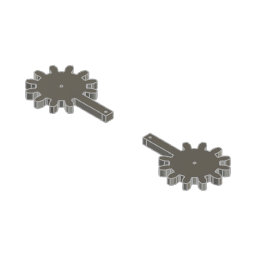
arm_gears v1 (Autodesk Fusion 360 design; units mm, degrees)
description: Spur Gear; Module: 5.0; Num Teeth: 12; Pressure Angle: 14.500000000000002; Backlash: 0.00 mm
Autodesk Fusion 360 part; units mm, degrees
(part 1 of 2)
sketch "スケッチ1" plane through (0, 0, 0) normal (0, 0, 1) x (1, 0, 0) in component "Spur Gear (12 teeth)"
  circle A0 centre (0, 0) radius 23.9492
  circle A1 centre (0, 0) radius 1.5
extrude "押し出し1" add sketch "スケッチ1" along normal blind 8 makes body 1 in component "Spur Gear (12 teeth)"
sketch "スケッチ2" plane through (0, 0, 0) normal (0, 0, 1) x (1, 0, 0) in component "Spur Gear (12 teeth)"
  spline S0 degree 5 poles (28.7745, -3.9507) (28.792, -3.9531) (28.8272, -3.9574) (28.88, -3.9623) (28.9507, -3.9658) (29.0393, -3.9662) (29.1282, -3.9638) (29.2172, -3.9595) (29.3063, -3.9544) (29.3954, -3.9485) (29.4846, -3.9419) (29.5738, -3.9345) (29.663, -3.9257) (29.7523, -3.9156) (29.8417, -3.904) (29.9311, -3.8911) (30.0205, -3.8771) (30.11, -3.8622) (30.1994, -3.8464) (30.2888, -3.8299) (30.3782, -3.8126) (30.4676, -3.7945) (30.557, -3.7754) (30.6464, -3.7555) (30.7357, -3.7347) (30.8251, -3.7131) (30.9144, -3.6907) (31.0037, -3.6675) (31.0929, -3.6435) (31.1821, -3.6189) (31.2712, -3.5935) (31.3604, -3.5674) (31.4494, -3.5406) (31.5384, -3.5131) (31.6274, -3.4848) (31.7163, -3.4559) (31.8051, -3.4263) (31.8939, -3.396) (31.9826, -3.365) (32.0713, -3.3335) (32.1598, -3.3012) (32.2484, -3.2683) (32.3368, -3.2348) (32.4251, -3.2007) (32.5134, -3.1659) (32.6016, -3.1305) (32.6897, -3.0945) (32.7778, -3.0579) (32.8657, -3.0207) (32.9536, -2.9829) (33.0413, -2.9445) (33.129, -2.9056) (33.2166, -2.866) (33.3041, -2.8259) (33.3915, -2.7852) (33.4787, -2.7439) (33.5659, -2.7021) (33.653, -2.6597) (33.7399, -2.6167) (33.8268, -2.5732) (33.9135, -2.5292) (34.0002, -2.4846) (34.0867, -2.4394) (34.1731, -2.3938) (34.2594, -2.3476) (34.3455, -2.3008) (34.4316, -2.2536) (34.5175, -2.2058) (34.6033, -2.1575) (34.6889, -2.1087) (34.7745, -2.0593) (34.8428, -2.0194) (34.894, -1.9893) (34.9281, -1.9691) (34.9451, -1.959) knots 0 0 0 0 0 0 0.01428571 0.02857143 0.04285714 0.05714286 0.07142857 0.08571429 0.1 0.11428571 0.12857143 0.14285714 0.15714286 0.17142857 0.18571429 0.2 0.21428571 0.22857143 0.24285714 0.25714286 0.27142857 0.28571429 0.3 0.31428571 0.32857143 0.34285714 0.35714286 0.37142857 0.38571429 0.4 0.41428571 0.42857143 0.44285714 0.45714286 0.47142857 0.48571429 0.5 0.51428571 0.52857143 0.54285714 0.55714286 0.57142857 0.58571429 0.6 0.61428571 0.62857143 0.64285714 0.65714286 0.67142857 0.68571429 0.7 0.71428571 0.72857143 0.74285714 0.75714286 0.77142857 0.78571429 0.8 0.81428571 0.82857143 0.84285714 0.85714286 0.87142857 0.88571429 0.9 0.91428571 0.92857143 0.94285714 0.95714286 0.97142857 0.98571429 1 1 1 1 1 1
  spline S1 degree 5 poles (28.7745, 3.9507) (28.792, 3.9531) (28.8272, 3.9574) (28.88, 3.9623) (28.9507, 3.9658) (29.0393, 3.9662) (29.1282, 3.9638) (29.2172, 3.9595) (29.3063, 3.9544) (29.3954, 3.9485) (29.4846, 3.9419) (29.5738, 3.9345) (29.663, 3.9257) (29.7523, 3.9156) (29.8417, 3.904) (29.9311, 3.8911) (30.0205, 3.8771) (30.11, 3.8622) (30.1994, 3.8464) (30.2888, 3.8299) (30.3782, 3.8126) (30.4676, 3.7945) (30.557, 3.7754) (30.6464, 3.7555) (30.7357, 3.7347) (30.8251, 3.7131) (30.9144, 3.6907) (31.0037, 3.6675) (31.0929, 3.6435) (31.1821, 3.6189) (31.2712, 3.5935) (31.3604, 3.5674) (31.4494, 3.5406) (31.5384, 3.5131) (31.6274, 3.4848) (31.7163, 3.4559) (31.8051, 3.4263) (31.8939, 3.396) (31.9826, 3.365) (32.0713, 3.3335) (32.1598, 3.3012) (32.2484, 3.2683) (32.3368, 3.2348) (32.4251, 3.2007) (32.5134, 3.1659) (32.6016, 3.1305) (32.6897, 3.0945) (32.7778, 3.0579) (32.8657, 3.0207) (32.9536, 2.9829) (33.0413, 2.9445) (33.129, 2.9056) (33.2166, 2.866) (33.3041, 2.8259) (33.3915, 2.7852) (33.4787, 2.7439) (33.5659, 2.7021) (33.653, 2.6597) (33.7399, 2.6167) (33.8268, 2.5732) (33.9135, 2.5292) (34.0002, 2.4846) (34.0867, 2.4394) (34.1731, 2.3938) (34.2594, 2.3476) (34.3455, 2.3008) (34.4316, 2.2536) (34.5175, 2.2058) (34.6033, 2.1575) (34.6889, 2.1087) (34.7745, 2.0593) (34.8428, 2.0194) (34.894, 1.9893) (34.9281, 1.9691) (34.9451, 1.959) knots 0 0 0 0 0 0 0.01428571 0.02857143 0.04285714 0.05714286 0.07142857 0.08571429 0.1 0.11428571 0.12857143 0.14285714 0.15714286 0.17142857 0.18571429 0.2 0.21428571 0.22857143 0.24285714 0.25714286 0.27142857 0.28571429 0.3 0.31428571 0.32857143 0.34285714 0.35714286 0.37142857 0.38571429 0.4 0.41428571 0.42857143 0.44285714 0.45714286 0.47142857 0.48571429 0.5 0.51428571 0.52857143 0.54285714 0.55714286 0.57142857 0.58571429 0.6 0.61428571 0.62857143 0.64285714 0.65714286 0.67142857 0.68571429 0.7 0.71428571 0.72857143 0.74285714 0.75714286 0.77142857 0.78571429 0.8 0.81428571 0.82857143 0.84285714 0.85714286 0.87142857 0.88571429 0.9 0.91428571 0.92857143 0.94285714 0.95714286 0.97142857 0.98571429 1 1 1 1 1 1
  arc A0 (34.9451, -1.959) -> (34.9451, 1.959) centre (0, 0) ccw
  line L0 (23.7167, -3.2576) -> (28.7745, -3.9507)
  line L1 (23.7167, 3.2576) -> (28.7745, 3.9507)
  line L2 (23.7167, -3.2576) -> (23.7167, 3.2576)
  point P0 (29.2025, -3.9601)
  point P1 (29.636, -3.9282)
  point P2 (30.0729, -3.8683)
  point P3 (30.5122, -3.7849)
  point P4 (30.9534, -3.6804)
  point P5 (31.396, -3.5566)
  point P6 (31.8397, -3.4144)
  point P7 (32.284, -3.2548)
  point P8 (32.7286, -3.0783)
  point P9 (33.1731, -2.8856)
  point P10 (33.6174, -2.6769)
  point P11 (34.061, -2.4528)
  point P12 (34.5037, -2.2134)
  point P13 (29.2025, 3.9601)
  point P14 (29.636, 3.9282)
  point P15 (30.0729, 3.8683)
  point P16 (30.5122, 3.7849)
  point P17 (30.9534, 3.6804)
  point P18 (31.396, 3.5566)
  point P19 (31.8397, 3.4144)
  point P20 (32.284, 3.2548)
  point P21 (32.7286, 3.0783)
  point P22 (33.1731, 2.8856)
  point P23 (33.6174, 2.6769)
  point P24 (34.061, 2.4528)
  point P25 (34.5037, 2.2134)
extrude "押し出し2" add sketch "スケッチ2" along normal blind 8 bodies 1 in component "Spur Gear (12 teeth)"
fillet "フィレット1" radius 1 2 edges at (23.7264, -3.2589, 4) (23.7264, 3.2589, 4) on bodies 1 in component "Spur Gear (12 teeth)"
pattern_circular "C パターン1" count 12 over 360 about axis through (0, 0, 0) along (0, 0, 1) of "押し出し2", "フィレット1" in component "Spur Gear (12 teeth)"
sketch "スケッチ3" plane through (0, 0, 0) normal (0, 0, 1) x (1, 0, 0) in component "Spur Gear (12 teeth)"
  circle A0 centre (0, 0) radius 30 construction
sketch "スケッチ1 (2)" plane through (0, 0, 8) normal (0, 0, 1) x (-1, 0, 0)
  arc A0 (-22.5216, 8.145) -> (-23.5768, 4.207) centre (0, 0) ccw
  arc A1 (-24.697, 3.3919) -> (-23.5768, 4.207) centre (-24.5612, 4.3827) ccw
  line L0 (-24.697, 3.3919) -> (-28.7745, 3.9507)
  spline S0 degree 5 poles (-28.7745, 3.9507) (-28.792, 3.9531) (-28.8272, 3.9574) (-28.88, 3.9623) (-28.9507, 3.9658) (-29.0393, 3.9662) (-29.1282, 3.9638) (-29.2172, 3.9595) (-29.3063, 3.9544) (-29.3954, 3.9485) (-29.4846, 3.9419) (-29.5738, 3.9345) (-29.663, 3.9257) (-29.7523, 3.9156) (-29.8417, 3.904) (-29.9311, 3.8911) (-30.0205, 3.8771) (-30.11, 3.8622) (-30.1994, 3.8464) (-30.2888, 3.8299) (-30.3782, 3.8126) (-30.4676, 3.7945) (-30.557, 3.7754) (-30.6464, 3.7555) (-30.7357, 3.7347) (-30.8251, 3.7131) (-30.9144, 3.6907) (-31.0037, 3.6675) (-31.0929, 3.6435) (-31.1821, 3.6189) (-31.2712, 3.5935) (-31.3604, 3.5674) (-31.4494, 3.5406) (-31.5384, 3.5131) (-31.6274, 3.4848) (-31.7163, 3.4559) (-31.8051, 3.4263) (-31.8939, 3.396) (-31.9826, 3.365) (-32.0713, 3.3335) (-32.1598, 3.3012) (-32.2484, 3.2683) (-32.3368, 3.2348) (-32.4251, 3.2007) (-32.5134, 3.1659) (-32.6016, 3.1305) (-32.6897, 3.0945) (-32.7778, 3.0579) (-32.8657, 3.0207) (-32.9536, 2.9829) (-33.0413, 2.9445) (-33.129, 2.9056) (-33.2166, 2.866) (-33.3041, 2.8259) (-33.3915, 2.7852) (-33.4787, 2.7439) (-33.5659, 2.7021) (-33.653, 2.6597) (-33.7399, 2.6167) (-33.8268, 2.5732) (-33.9135, 2.5292) (-34.0002, 2.4846) (-34.0867, 2.4394) (-34.1731, 2.3938) (-34.2594, 2.3476) (-34.3455, 2.3008) (-34.4316, 2.2536) (-34.5175, 2.2058) (-34.6033, 2.1575) (-34.6889, 2.1087) (-34.7745, 2.0593) (-34.8428, 2.0194) (-34.894, 1.9893) (-34.9281, 1.9691) (-34.9451, 1.959) knots 0 0 0 0 0 0 0.01428571 0.02857143 0.04285714 0.05714286 0.07142857 0.08571429 0.1 0.11428571 0.12857143 0.14285714 0.15714286 0.17142857 0.18571429 0.2 0.21428571 0.22857143 0.24285714 0.25714286 0.27142857 0.28571429 0.3 0.31428571 0.32857143 0.34285714 0.35714286 0.37142857 0.38571429 0.4 0.41428571 0.42857143 0.44285714 0.45714286 0.47142857 0.48571429 0.5 0.51428571 0.52857143 0.54285714 0.55714286 0.57142857 0.58571429 0.6 0.61428571 0.62857143 0.64285714 0.65714286 0.67142857 0.68571429 0.7 0.71428571 0.72857143 0.74285714 0.75714286 0.77142857 0.78571429 0.8 0.81428571 0.82857143 0.84285714 0.85714286 0.87142857 0.88571429 0.9 0.91428571 0.92857143 0.94285714 0.95714286 0.97142857 0.98571429 1 1 1 1 1 1
  arc A2 (-34.9451, 1.959) -> (-34.9451, -1.959) centre (0, 0) ccw
  spline S1 degree 5 poles (-34.9451, -1.959) (-34.9281, -1.9691) (-34.894, -1.9893) (-34.8428, -2.0194) (-34.7745, -2.0593) (-34.6889, -2.1087) (-34.6033, -2.1575) (-34.5175, -2.2058) (-34.4316, -2.2536) (-34.3455, -2.3008) (-34.2594, -2.3476) (-34.1731, -2.3938) (-34.0867, -2.4394) (-34.0002, -2.4846) (-33.9135, -2.5292) (-33.8268, -2.5732) (-33.7399, -2.6167) (-33.653, -2.6597) (-33.5659, -2.7021) (-33.4787, -2.7439) (-33.3915, -2.7852) (-33.3041, -2.8259) (-33.2166, -2.866) (-33.129, -2.9056) (-33.0413, -2.9445) (-32.9536, -2.9829) (-32.8657, -3.0207) (-32.7778, -3.0579) (-32.6897, -3.0945) (-32.6016, -3.1305) (-32.5134, -3.1659) (-32.4251, -3.2007) (-32.3368, -3.2348) (-32.2484, -3.2683) (-32.1598, -3.3012) (-32.0713, -3.3335) (-31.9826, -3.365) (-31.8939, -3.396) (-31.8051, -3.4263) (-31.7163, -3.4559) (-31.6274, -3.4848) (-31.5384, -3.5131) (-31.4494, -3.5406) (-31.3604, -3.5674) (-31.2712, -3.5935) (-31.1821, -3.6189) (-31.0929, -3.6435) (-31.0037, -3.6675) (-30.9144, -3.6907) (-30.8251, -3.7131) (-30.7357, -3.7347) (-30.6464, -3.7555) (-30.557, -3.7754) (-30.4676, -3.7945) (-30.3782, -3.8126) (-30.2888, -3.8299) (-30.1994, -3.8464) (-30.11, -3.8622) (-30.0205, -3.8771) (-29.9311, -3.8911) (-29.8417, -3.904) (-29.7523, -3.9156) (-29.663, -3.9257) (-29.5738, -3.9345) (-29.4846, -3.9419) (-29.3954, -3.9485) (-29.3063, -3.9544) (-29.2172, -3.9595) (-29.1282, -3.9638) (-29.0393, -3.9662) (-28.9507, -3.9658) (-28.88, -3.9623) (-28.8272, -3.9574) (-28.792, -3.9531) (-28.7745, -3.9507) knots -1 -1 -1 -1 -1 -1 -0.98571429 -0.97142857 -0.95714286 -0.94285714 -0.92857143 -0.91428571 -0.9 -0.88571429 -0.87142857 -0.85714286 -0.84285714 -0.82857143 -0.81428571 -0.8 -0.78571429 -0.77142857 -0.75714286 -0.74285714 -0.72857143 -0.71428571 -0.7 -0.68571429 -0.67142857 -0.65714286 -0.64285714 -0.62857143 -0.61428571 -0.6 -0.58571429 -0.57142857 -0.55714286 -0.54285714 -0.52857143 -0.51428571 -0.5 -0.48571429 -0.47142857 -0.45714286 -0.44285714 -0.42857143 -0.41428571 -0.4 -0.38571429 -0.37142857 -0.35714286 -0.34285714 -0.32857143 -0.31428571 -0.3 -0.28571429 -0.27142857 -0.25714286 -0.24285714 -0.22857143 -0.21428571 -0.2 -0.18571429 -0.17142857 -0.15714286 -0.14285714 -0.12857143 -0.11428571 -0.1 -0.08571429 -0.07142857 -0.05714286 -0.04285714 -0.02857143 -0.01428571 0 0 0 0 0 0
  line L1 (-28.7745, -3.9507) -> (-24.697, -3.3919)
  arc A3 (-23.5768, -4.207) -> (-24.697, -3.3919) centre (-24.5612, -4.3827) ccw
  arc A4 (-23.5768, -4.207) -> (-22.5216, -8.145) centre (0, 0) ccw
  arc A5 (-23.0842, -9.411) -> (-22.5216, -8.145) centre (-23.462, -8.4851) ccw
  line L2 (-23.0842, -9.411) -> (-26.8948, -10.9659)
  spline S2 degree 5 poles (-26.8948, -10.9659) (-26.9112, -10.9726) (-26.9438, -10.9864) (-26.992, -11.0086) (-27.055, -11.0409) (-27.1319, -11.0848) (-27.2076, -11.1314) (-27.2826, -11.1795) (-27.3571, -11.2286) (-27.4314, -11.2782) (-27.5053, -11.3285) (-27.5789, -11.3795) (-27.6518, -11.4317) (-27.7241, -11.4852) (-27.7957, -11.5399) (-27.8667, -11.5957) (-27.9371, -11.6526) (-28.0071, -11.7102) (-28.0767, -11.7686) (-28.1458, -11.8276) (-28.2146, -11.8873) (-28.283, -11.9477) (-28.3509, -12.0089) (-28.4183, -12.0708) (-28.4853, -12.1335) (-28.5519, -12.1969) (-28.618, -12.261) (-28.6837, -12.3257) (-28.749, -12.3911) (-28.8139, -12.457) (-28.8784, -12.5236) (-28.9426, -12.5907) (-29.0063, -12.6585) (-29.0696, -12.7268) (-29.1325, -12.7958) (-29.195, -12.8653) (-29.2572, -12.9353) (-29.3189, -13.0059) (-29.3803, -13.0771) (-29.4413, -13.1488) (-29.5019, -13.221) (-29.5621, -13.2937) (-29.6219, -13.367) (-29.6813, -13.4407) (-29.7404, -13.515) (-29.7991, -13.5897) (-29.8574, -13.6649) (-29.9154, -13.7406) (-29.9729, -13.8168) (-30.0301, -13.8935) (-30.0869, -13.9706) (-30.1434, -14.0482) (-30.1994, -14.1263) (-30.2551, -14.2048) (-30.3104, -14.2837) (-30.3654, -14.3631) (-30.42, -14.4429) (-30.4742, -14.5231) (-30.528, -14.6038) (-30.5815, -14.6849) (-30.6346, -14.7664) (-30.6873, -14.8484) (-30.7397, -14.9307) (-30.7916, -15.0135) (-30.8433, -15.0966) (-30.8945, -15.1802) (-30.9454, -15.2641) (-30.9959, -15.3485) (-31.0461, -15.4332) (-31.0958, -15.5183) (-31.1452, -15.6038) (-31.1845, -15.6725) (-31.2137, -15.7242) (-31.2332, -15.7587) (-31.2429, -15.776) knots 0 0 0 0 0 0 0.01428571 0.02857143 0.04285714 0.05714286 0.07142857 0.08571429 0.1 0.11428571 0.12857143 0.14285714 0.15714286 0.17142857 0.18571429 0.2 0.21428571 0.22857143 0.24285714 0.25714286 0.27142857 0.28571429 0.3 0.31428571 0.32857143 0.34285714 0.35714286 0.37142857 0.38571429 0.4 0.41428571 0.42857143 0.44285714 0.45714286 0.47142857 0.48571429 0.5 0.51428571 0.52857143 0.54285714 0.55714286 0.57142857 0.58571429 0.6 0.61428571 0.62857143 0.64285714 0.65714286 0.67142857 0.68571429 0.7 0.71428571 0.72857143 0.74285714 0.75714286 0.77142857 0.78571429 0.8 0.81428571 0.82857143 0.84285714 0.85714286 0.87142857 0.88571429 0.9 0.91428571 0.92857143 0.94285714 0.95714286 0.97142857 0.98571429 1 1 1 1 1 1
  arc A6 (-31.2429, -15.776) -> (-29.2839, -19.1691) centre (0, 0) ccw
  spline S3 degree 5 poles (-29.2839, -19.1691) (-29.2641, -19.1693) (-29.2244, -19.1698) (-29.165, -19.1703) (-29.0859, -19.1707) (-28.9872, -19.1706) (-28.8886, -19.1701) (-28.7901, -19.169) (-28.6918, -19.1674) (-28.5937, -19.1653) (-28.4957, -19.1627) (-28.3979, -19.1596) (-28.3002, -19.156) (-28.2027, -19.1518) (-28.1054, -19.1471) (-28.0082, -19.1419) (-27.9113, -19.1361) (-27.8145, -19.1298) (-27.7179, -19.123) (-27.6215, -19.1157) (-27.5253, -19.1078) (-27.4292, -19.0993) (-27.3334, -19.0903) (-27.2378, -19.0808) (-27.1424, -19.0707) (-27.0472, -19.0601) (-26.9522, -19.0489) (-26.8574, -19.0371) (-26.7629, -19.0248) (-26.6686, -19.0119) (-26.5745, -18.9985) (-26.4807, -18.9844) (-26.3871, -18.9698) (-26.2937, -18.9546) (-26.2006, -18.9389) (-26.1078, -18.9225) (-26.0152, -18.9055) (-25.9229, -18.888) (-25.8309, -18.8698) (-25.7392, -18.851) (-25.6477, -18.8316) (-25.5565, -18.8116) (-25.4657, -18.7909) (-25.3752, -18.7696) (-25.2849, -18.7477) (-25.1951, -18.7251) (-25.1055, -18.7018) (-25.0162, -18.6779) (-24.9273, -18.6534) (-24.8388, -18.6282) (-24.7506, -18.6022) (-24.6628, -18.5756) (-24.5754, -18.5481) (-24.4885, -18.5199) (-24.402, -18.4909) (-24.3159, -18.4612) (-24.2302, -18.4308) (-24.1449, -18.3997) (-24.06, -18.3679) (-23.9755, -18.3354) (-23.8917, -18.3018) (-23.8085, -18.2672) (-23.7261, -18.2313) (-23.6444, -18.1942) (-23.5634, -18.1561) (-23.4829, -18.1172) (-23.4028, -18.0777) (-23.3231, -18.0377) (-23.2439, -17.9968) (-23.1657, -17.9545) (-23.0891, -17.9099) (-23.0297, -17.8714) (-22.9864, -17.8408) (-22.9581, -17.8195) (-22.9441, -17.8086) knots -1 -1 -1 -1 -1 -1 -0.98571429 -0.97142857 -0.95714286 -0.94285714 -0.92857143 -0.91428571 -0.9 -0.88571429 -0.87142857 -0.85714286 -0.84285714 -0.82857143 -0.81428571 -0.8 -0.78571429 -0.77142857 -0.75714286 -0.74285714 -0.72857143 -0.71428571 -0.7 -0.68571429 -0.67142857 -0.65714286 -0.64285714 -0.62857143 -0.61428571 -0.6 -0.58571429 -0.57142857 -0.55714286 -0.54285714 -0.52857143 -0.51428571 -0.5 -0.48571429 -0.47142857 -0.45714286 -0.44285714 -0.42857143 -0.41428571 -0.4 -0.38571429 -0.37142857 -0.35714286 -0.34285714 -0.32857143 -0.31428571 -0.3 -0.28571429 -0.27142857 -0.25714286 -0.24285714 -0.22857143 -0.21428571 -0.2 -0.18571429 -0.17142857 -0.15714286 -0.14285714 -0.12857143 -0.11428571 -0.1 -0.08571429 -0.07142857 -0.05714286 -0.04285714 -0.02857143 -0.01428571 0 0 0 0 0 0
  line L3 (-22.9441, -17.8086) -> (-19.6923, -15.286)
  arc A7 (-18.3146, -15.4318) -> (-19.6923, -15.286) centre (-19.0793, -16.0761) ccw
  arc A8 (-18.3146, -15.4318) -> (-15.4318, -18.3146) centre (0, 0) ccw
  arc A9 (-15.286, -19.6923) -> (-15.4318, -18.3146) centre (-16.0761, -19.0793) ccw
  line L4 (-15.286, -19.6923) -> (-17.8086, -22.9441)
  spline S4 degree 5 poles (-17.8086, -22.9441) (-17.8195, -22.9581) (-17.8408, -22.9864) (-17.8714, -23.0297) (-17.9099, -23.0891) (-17.9545, -23.1657) (-17.9968, -23.2439) (-18.0377, -23.3231) (-18.0777, -23.4028) (-18.1172, -23.4829) (-18.1561, -23.5634) (-18.1942, -23.6444) (-18.2313, -23.7261) (-18.2672, -23.8085) (-18.3018, -23.8917) (-18.3354, -23.9755) (-18.3679, -24.06) (-18.3997, -24.1449) (-18.4308, -24.2302) (-18.4612, -24.3159) (-18.4909, -24.402) (-18.5199, -24.4885) (-18.5481, -24.5754) (-18.5756, -24.6628) (-18.6022, -24.7506) (-18.6282, -24.8388) (-18.6534, -24.9273) (-18.6779, -25.0162) (-18.7018, -25.1055) (-18.7251, -25.1951) (-18.7477, -25.2849) (-18.7696, -25.3752) (-18.7909, -25.4657) (-18.8116, -25.5565) (-18.8316, -25.6477) (-18.851, -25.7392) (-18.8698, -25.8309) (-18.888, -25.9229) (-18.9055, -26.0152) (-18.9225, -26.1078) (-18.9389, -26.2006) (-18.9546, -26.2937) (-18.9698, -26.3871) (-18.9844, -26.4807) (-18.9985, -26.5745) (-19.0119, -26.6686) (-19.0248, -26.7629) (-19.0371, -26.8574) (-19.0489, -26.9522) (-19.0601, -27.0472) (-19.0707, -27.1424) (-19.0808, -27.2378) (-19.0903, -27.3334) (-19.0993, -27.4292) (-19.1078, -27.5253) (-19.1157, -27.6215) (-19.123, -27.7179) (-19.1298, -27.8145) (-19.1361, -27.9113) (-19.1419, -28.0082) (-19.1471, -28.1054) (-19.1518, -28.2027) (-19.156, -28.3002) (-19.1596, -28.3979) (-19.1627, -28.4957) (-19.1653, -28.5937) (-19.1674, -28.6918) (-19.169, -28.7901) (-19.1701, -28.8886) (-19.1706, -28.9872) (-19.1707, -29.0859) (-19.1703, -29.165) (-19.1698, -29.2244) (-19.1693, -29.2641) (-19.1691, -29.2839) knots 0 0 0 0 0 0 0.01428571 0.02857143 0.04285714 0.05714286 0.07142857 0.08571429 0.1 0.11428571 0.12857143 0.14285714 0.15714286 0.17142857 0.18571429 0.2 0.21428571 0.22857143 0.24285714 0.25714286 0.27142857 0.28571429 0.3 0.31428571 0.32857143 0.34285714 0.35714286 0.37142857 0.38571429 0.4 0.41428571 0.42857143 0.44285714 0.45714286 0.47142857 0.48571429 0.5 0.51428571 0.52857143 0.54285714 0.55714286 0.57142857 0.58571429 0.6 0.61428571 0.62857143 0.64285714 0.65714286 0.67142857 0.68571429 0.7 0.71428571 0.72857143 0.74285714 0.75714286 0.77142857 0.78571429 0.8 0.81428571 0.82857143 0.84285714 0.85714286 0.87142857 0.88571429 0.9 0.91428571 0.92857143 0.94285714 0.95714286 0.97142857 0.98571429 1 1 1 1 1 1
  arc A10 (-19.1691, -29.2839) -> (-15.776, -31.2429) centre (0, 0) ccw
  spline S5 degree 5 poles (-15.776, -31.2429) (-15.7587, -31.2332) (-15.7242, -31.2137) (-15.6725, -31.1845) (-15.6038, -31.1452) (-15.5183, -31.0958) (-15.4332, -31.0461) (-15.3485, -30.9959) (-15.2641, -30.9454) (-15.1802, -30.8945) (-15.0966, -30.8433) (-15.0135, -30.7916) (-14.9307, -30.7397) (-14.8484, -30.6873) (-14.7664, -30.6346) (-14.6849, -30.5815) (-14.6038, -30.528) (-14.5231, -30.4742) (-14.4429, -30.42) (-14.3631, -30.3654) (-14.2837, -30.3104) (-14.2048, -30.2551) (-14.1263, -30.1994) (-14.0482, -30.1434) (-13.9706, -30.0869) (-13.8935, -30.0301) (-13.8168, -29.9729) (-13.7406, -29.9154) (-13.6649, -29.8574) (-13.5897, -29.7991) (-13.515, -29.7404) (-13.4407, -29.6813) (-13.367, -29.6219) (-13.2937, -29.5621) (-13.221, -29.5019) (-13.1488, -29.4413) (-13.0771, -29.3803) (-13.0059, -29.3189) (-12.9353, -29.2572) (-12.8653, -29.195) (-12.7958, -29.1325) (-12.7268, -29.0696) (-12.6585, -29.0063) (-12.5907, -28.9426) (-12.5236, -28.8784) (-12.457, -28.8139) (-12.3911, -28.749) (-12.3257, -28.6837) (-12.261, -28.618) (-12.1969, -28.5519) (-12.1335, -28.4853) (-12.0708, -28.4183) (-12.0089, -28.3509) (-11.9477, -28.283) (-11.8873, -28.2146) (-11.8276, -28.1458) (-11.7686, -28.0767) (-11.7102, -28.0071) (-11.6526, -27.9371) (-11.5957, -27.8667) (-11.5399, -27.7957) (-11.4852, -27.7241) (-11.4317, -27.6518) (-11.3795, -27.5789) (-11.3285, -27.5053) (-11.2782, -27.4314) (-11.2286, -27.3571) (-11.1795, -27.2826) (-11.1314, -27.2076) (-11.0848, -27.1319) (-11.0409, -27.055) (-11.0086, -26.992) (-10.9864, -26.9438) (-10.9726, -26.9112) (-10.9659, -26.8948) knots -1 -1 -1 -1 -1 -1 -0.98571429 -0.97142857 -0.95714286 -0.94285714 -0.92857143 -0.91428571 -0.9 -0.88571429 -0.87142857 -0.85714286 -0.84285714 -0.82857143 -0.81428571 -0.8 -0.78571429 -0.77142857 -0.75714286 -0.74285714 -0.72857143 -0.71428571 -0.7 -0.68571429 -0.67142857 -0.65714286 -0.64285714 -0.62857143 -0.61428571 -0.6 -0.58571429 -0.57142857 -0.55714286 -0.54285714 -0.52857143 -0.51428571 -0.5 -0.48571429 -0.47142857 -0.45714286 -0.44285714 -0.42857143 -0.41428571 -0.4 -0.38571429 -0.37142857 -0.35714286 -0.34285714 -0.32857143 -0.31428571 -0.3 -0.28571429 -0.27142857 -0.25714286 -0.24285714 -0.22857143 -0.21428571 -0.2 -0.18571429 -0.17142857 -0.15714286 -0.14285714 -0.12857143 -0.11428571 -0.1 -0.08571429 -0.07142857 -0.05714286 -0.04285714 -0.02857143 -0.01428571 0 0 0 0 0 0
  line L5 (-10.9659, -26.8948) -> (-9.411, -23.0842)
  arc A11 (-8.145, -22.5216) -> (-9.411, -23.0842) centre (-8.4851, -23.462) ccw
  arc A12 (-8.145, -22.5216) -> (-4.207, -23.5768) centre (0, 0) ccw
  arc A13 (-3.3919, -24.697) -> (-4.207, -23.5768) centre (-4.3827, -24.5612) ccw
  line L6 (-3.3919, -24.697) -> (-3.9507, -28.7745)
  spline S6 degree 5 poles (-3.9507, -28.7745) (-3.9531, -28.792) (-3.9574, -28.8272) (-3.9623, -28.88) (-3.9658, -28.9507) (-3.9662, -29.0393) (-3.9638, -29.1282) (-3.9595, -29.2172) (-3.9544, -29.3063) (-3.9485, -29.3954) (-3.9419, -29.4846) (-3.9345, -29.5738) (-3.9257, -29.663) (-3.9156, -29.7523) (-3.904, -29.8417) (-3.8911, -29.9311) (-3.8771, -30.0205) (-3.8622, -30.11) (-3.8464, -30.1994) (-3.8299, -30.2888) (-3.8126, -30.3782) (-3.7945, -30.4676) (-3.7754, -30.557) (-3.7555, -30.6464) (-3.7347, -30.7357) (-3.7131, -30.8251) (-3.6907, -30.9144) (-3.6675, -31.0037) (-3.6435, -31.0929) (-3.6189, -31.1821) (-3.5935, -31.2712) (-3.5674, -31.3604) (-3.5406, -31.4494) (-3.5131, -31.5384) (-3.4848, -31.6274) (-3.4559, -31.7163) (-3.4263, -31.8051) (-3.396, -31.8939) (-3.365, -31.9826) (-3.3335, -32.0713) (-3.3012, -32.1598) (-3.2683, -32.2484) (-3.2348, -32.3368) (-3.2007, -32.4251) (-3.1659, -32.5134) (-3.1305, -32.6016) (-3.0945, -32.6897) (-3.0579, -32.7778) (-3.0207, -32.8657) (-2.9829, -32.9536) (-2.9445, -33.0413) (-2.9056, -33.129) (-2.866, -33.2166) (-2.8259, -33.3041) (-2.7852, -33.3915) (-2.7439, -33.4787) (-2.7021, -33.5659) (-2.6597, -33.653) (-2.6167, -33.7399) (-2.5732, -33.8268) (-2.5292, -33.9135) (-2.4846, -34.0002) (-2.4394, -34.0867) (-2.3938, -34.1731) (-2.3476, -34.2594) (-2.3008, -34.3455) (-2.2536, -34.4316) (-2.2058, -34.5175) (-2.1575, -34.6033) (-2.1087, -34.6889) (-2.0593, -34.7745) (-2.0194, -34.8428) (-1.9893, -34.894) (-1.9691, -34.9281) (-1.959, -34.9451) knots 0 0 0 0 0 0 0.01428571 0.02857143 0.04285714 0.05714286 0.07142857 0.08571429 0.1 0.11428571 0.12857143 0.14285714 0.15714286 0.17142857 0.18571429 0.2 0.21428571 0.22857143 0.24285714 0.25714286 0.27142857 0.28571429 0.3 0.31428571 0.32857143 0.34285714 0.35714286 0.37142857 0.38571429 0.4 0.41428571 0.42857143 0.44285714 0.45714286 0.47142857 0.48571429 0.5 0.51428571 0.52857143 0.54285714 0.55714286 0.57142857 0.58571429 0.6 0.61428571 0.62857143 0.64285714 0.65714286 0.67142857 0.68571429 0.7 0.71428571 0.72857143 0.74285714 0.75714286 0.77142857 0.78571429 0.8 0.81428571 0.82857143 0.84285714 0.85714286 0.87142857 0.88571429 0.9 0.91428571 0.92857143 0.94285714 0.95714286 0.97142857 0.98571429 1 1 1 1 1 1
  arc A14 (-1.959, -34.9451) -> (1.959, -34.9451) centre (0, 0) ccw
  spline S7 degree 5 poles (1.959, -34.9451) (1.9691, -34.9281) (1.9893, -34.894) (2.0194, -34.8428) (2.0593, -34.7745) (2.1087, -34.6889) (2.1575, -34.6033) (2.2058, -34.5175) (2.2536, -34.4316) (2.3008, -34.3455) (2.3476, -34.2594) (2.3938, -34.1731) (2.4394, -34.0867) (2.4846, -34.0002) (2.5292, -33.9135) (2.5732, -33.8268) (2.6167, -33.7399) (2.6597, -33.653) (2.7021, -33.5659) (2.7439, -33.4787) (2.7852, -33.3915) (2.8259, -33.3041) (2.866, -33.2166) (2.9056, -33.129) (2.9445, -33.0413) (2.9829, -32.9536) (3.0207, -32.8657) (3.0579, -32.7778) (3.0945, -32.6897) (3.1305, -32.6016) (3.1659, -32.5134) (3.2007, -32.4251) (3.2348, -32.3368) (3.2683, -32.2484) (3.3012, -32.1598) (3.3335, -32.0713) (3.365, -31.9826) (3.396, -31.8939) (3.4263, -31.8051) (3.4559, -31.7163) (3.4848, -31.6274) (3.5131, -31.5384) (3.5406, -31.4494) (3.5674, -31.3604) (3.5935, -31.2712) (3.6189, -31.1821) (3.6435, -31.0929) (3.6675, -31.0037) (3.6907, -30.9144) (3.7131, -30.8251) (3.7347, -30.7357) (3.7555, -30.6464) (3.7754, -30.557) (3.7945, -30.4676) (3.8126, -30.3782) (3.8299, -30.2888) (3.8464, -30.1994) (3.8622, -30.11) (3.8771, -30.0205) (3.8911, -29.9311) (3.904, -29.8417) (3.9156, -29.7523) (3.9257, -29.663) (3.9345, -29.5738) (3.9419, -29.4846) (3.9485, -29.3954) (3.9544, -29.3063) (3.9595, -29.2172) (3.9638, -29.1282) (3.9662, -29.0393) (3.9658, -28.9507) (3.9623, -28.88) (3.9574, -28.8272) (3.9531, -28.792) (3.9507, -28.7745) knots -1 -1 -1 -1 -1 -1 -0.98571429 -0.97142857 -0.95714286 -0.94285714 -0.92857143 -0.91428571 -0.9 -0.88571429 -0.87142857 -0.85714286 -0.84285714 -0.82857143 -0.81428571 -0.8 -0.78571429 -0.77142857 -0.75714286 -0.74285714 -0.72857143 -0.71428571 -0.7 -0.68571429 -0.67142857 -0.65714286 -0.64285714 -0.62857143 -0.61428571 -0.6 -0.58571429 -0.57142857 -0.55714286 -0.54285714 -0.52857143 -0.51428571 -0.5 -0.48571429 -0.47142857 -0.45714286 -0.44285714 -0.42857143 -0.41428571 -0.4 -0.38571429 -0.37142857 -0.35714286 -0.34285714 -0.32857143 -0.31428571 -0.3 -0.28571429 -0.27142857 -0.25714286 -0.24285714 -0.22857143 -0.21428571 -0.2 -0.18571429 -0.17142857 -0.15714286 -0.14285714 -0.12857143 -0.11428571 -0.1 -0.08571429 -0.07142857 -0.05714286 -0.04285714 -0.02857143 -0.01428571 0 0 0 0 0 0
  line L7 (3.9507, -28.7745) -> (3.3919, -24.697)
  arc A15 (4.207, -23.5768) -> (3.3919, -24.697) centre (4.3827, -24.5612) ccw
  arc A16 (4.207, -23.5768) -> (8.145, -22.5216) centre (0, 0) ccw
  arc A17 (9.411, -23.0842) -> (8.145, -22.5216) centre (8.4851, -23.462) ccw
  line L8 (9.411, -23.0842) -> (10.9659, -26.8948)
  spline S8 degree 5 poles (10.9659, -26.8948) (10.9726, -26.9112) (10.9864, -26.9438) (11.0086, -26.992) (11.0409, -27.055) (11.0848, -27.1319) (11.1314, -27.2076) (11.1795, -27.2826) (11.2286, -27.3571) (11.2782, -27.4314) (11.3285, -27.5053) (11.3795, -27.5789) (11.4317, -27.6518) (11.4852, -27.7241) (11.5399, -27.7957) (11.5957, -27.8667) (11.6526, -27.9371) (11.7102, -28.0071) (11.7686, -28.0767) (11.8276, -28.1458) (11.8873, -28.2146) (11.9477, -28.283) (12.0089, -28.3509) (12.0708, -28.4183) (12.1335, -28.4853) (12.1969, -28.5519) (12.261, -28.618) (12.3257, -28.6837) (12.3911, -28.749) (12.457, -28.8139) (12.5236, -28.8784) (12.5907, -28.9426) (12.6585, -29.0063) (12.7268, -29.0696) (12.7958, -29.1325) (12.8653, -29.195) (12.9353, -29.2572) (13.0059, -29.3189) (13.0771, -29.3803) (13.1488, -29.4413) (13.221, -29.5019) (13.2937, -29.5621) (13.367, -29.6219) (13.4407, -29.6813) (13.515, -29.7404) (13.5897, -29.7991) (13.6649, -29.8574) (13.7406, -29.9154) (13.8168, -29.9729) (13.8935, -30.0301) (13.9706, -30.0869) (14.0482, -30.1434) (14.1263, -30.1994) (14.2048, -30.2551) (14.2837, -30.3104) (14.3631, -30.3654) (14.4429, -30.42) (14.5231, -30.4742) (14.6038, -30.528) (14.6849, -30.5815) (14.7664, -30.6346) (14.8484, -30.6873) (14.9307, -30.7397) (15.0135, -30.7916) (15.0966, -30.8433) (15.1802, -30.8945) (15.2641, -30.9454) (15.3485, -30.9959) (15.4332, -31.0461) (15.5183, -31.0958) (15.6038, -31.1452) (15.6725, -31.1845) (15.7242, -31.2137) (15.7587, -31.2332) (15.776, -31.2429) knots 0 0 0 0 0 0 0.01428571 0.02857143 0.04285714 0.05714286 0.07142857 0.08571429 0.1 0.11428571 0.12857143 0.14285714 0.15714286 0.17142857 0.18571429 0.2 0.21428571 0.22857143 0.24285714 0.25714286 0.27142857 0.28571429 0.3 0.31428571 0.32857143 0.34285714 0.35714286 0.37142857 0.38571429 0.4 0.41428571 0.42857143 0.44285714 0.45714286 0.47142857 0.48571429 0.5 0.51428571 0.52857143 0.54285714 0.55714286 0.57142857 0.58571429 0.6 0.61428571 0.62857143 0.64285714 0.65714286 0.67142857 0.68571429 0.7 0.71428571 0.72857143 0.74285714 0.75714286 0.77142857 0.78571429 0.8 0.81428571 0.82857143 0.84285714 0.85714286 0.87142857 0.88571429 0.9 0.91428571 0.92857143 0.94285714 0.95714286 0.97142857 0.98571429 1 1 1 1 1 1
  arc A18 (15.776, -31.2429) -> (19.1691, -29.2839) centre (0, 0) ccw
  spline S9 degree 5 poles (19.1691, -29.2839) (19.1693, -29.2641) (19.1698, -29.2244) (19.1703, -29.165) (19.1707, -29.0859) (19.1706, -28.9872) (19.1701, -28.8886) (19.169, -28.7901) (19.1674, -28.6918) (19.1653, -28.5937) (19.1627, -28.4957) (19.1596, -28.3979) (19.156, -28.3002) (19.1518, -28.2027) (19.1471, -28.1054) (19.1419, -28.0082) (19.1361, -27.9113) (19.1298, -27.8145) (19.123, -27.7179) (19.1157, -27.6215) (19.1078, -27.5253) (19.0993, -27.4292) (19.0903, -27.3334) (19.0808, -27.2378) (19.0707, -27.1424) (19.0601, -27.0472) (19.0489, -26.9522) (19.0371, -26.8574) (19.0248, -26.7629) (19.0119, -26.6686) (18.9985, -26.5745) (18.9844, -26.4807) (18.9698, -26.3871) (18.9546, -26.2937) (18.9389, -26.2006) (18.9225, -26.1078) (18.9055, -26.0152) (18.888, -25.9229) (18.8698, -25.8309) (18.851, -25.7392) (18.8316, -25.6477) (18.8116, -25.5565) (18.7909, -25.4657) (18.7696, -25.3752) (18.7477, -25.2849) (18.7251, -25.1951) (18.7018, -25.1055) (18.6779, -25.0162) (18.6534, -24.9273) (18.6282, -24.8388) (18.6022, -24.7506) (18.5756, -24.6628) (18.5481, -24.5754) (18.5199, -24.4885) (18.4909, -24.402) (18.4612, -24.3159) (18.4308, -24.2302) (18.3997, -24.1449) (18.3679, -24.06) (18.3354, -23.9755) (18.3018, -23.8917) (18.2672, -23.8085) (18.2313, -23.7261) (18.1942, -23.6444) (18.1561, -23.5634) (18.1172, -23.4829) (18.0777, -23.4028) (18.0377, -23.3231) (17.9968, -23.2439) (17.9545, -23.1657) (17.9099, -23.0891) (17.8714, -23.0297) (17.8408, -22.9864) (17.8195, -22.9581) (17.8086, -22.9441) knots -1 -1 -1 -1 -1 -1 -0.98571429 -0.97142857 -0.95714286 -0.94285714 -0.92857143 -0.91428571 -0.9 -0.88571429 -0.87142857 -0.85714286 -0.84285714 -0.82857143 -0.81428571 -0.8 -0.78571429 -0.77142857 -0.75714286 -0.74285714 -0.72857143 -0.71428571 -0.7 -0.68571429 -0.67142857 -0.65714286 -0.64285714 -0.62857143 -0.61428571 -0.6 -0.58571429 -0.57142857 -0.55714286 -0.54285714 -0.52857143 -0.51428571 -0.5 -0.48571429 -0.47142857 -0.45714286 -0.44285714 -0.42857143 -0.41428571 -0.4 -0.38571429 -0.37142857 -0.35714286 -0.34285714 -0.32857143 -0.31428571 -0.3 -0.28571429 -0.27142857 -0.25714286 -0.24285714 -0.22857143 -0.21428571 -0.2 -0.18571429 -0.17142857 -0.15714286 -0.14285714 -0.12857143 -0.11428571 -0.1 -0.08571429 -0.07142857 -0.05714286 -0.04285714 -0.02857143 -0.01428571 0 0 0 0 0 0
  line L9 (17.8086, -22.9441) -> (15.286, -19.6923)
  arc A19 (15.4318, -18.3146) -> (15.286, -19.6923) centre (16.0761, -19.0793) ccw
  arc A20 (15.4318, -18.3146) -> (18.3146, -15.4318) centre (0, 0) ccw
  arc A21 (19.6923, -15.286) -> (18.3146, -15.4318) centre (19.0793, -16.0761) ccw
  line L10 (19.6923, -15.286) -> (22.9441, -17.8086)
  spline S10 degree 5 poles (22.9441, -17.8086) (22.9581, -17.8195) (22.9864, -17.8408) (23.0297, -17.8714) (23.0891, -17.9099) (23.1657, -17.9545) (23.2439, -17.9968) (23.3231, -18.0377) (23.4028, -18.0777) (23.4829, -18.1172) (23.5634, -18.1561) (23.6444, -18.1942) (23.7261, -18.2313) (23.8085, -18.2672) (23.8917, -18.3018) (23.9755, -18.3354) (24.06, -18.3679) (24.1449, -18.3997) (24.2302, -18.4308) (24.3159, -18.4612) (24.402, -18.4909) (24.4885, -18.5199) (24.5754, -18.5481) (24.6628, -18.5756) (24.7506, -18.6022) (24.8388, -18.6282) (24.9273, -18.6534) (25.0162, -18.6779) (25.1055, -18.7018) (25.1951, -18.7251) (25.2849, -18.7477) (25.3752, -18.7696) (25.4657, -18.7909) (25.5565, -18.8116) (25.6477, -18.8316) (25.7392, -18.851) (25.8309, -18.8698) (25.9229, -18.888) (26.0152, -18.9055) (26.1078, -18.9225) (26.2006, -18.9389) (26.2937, -18.9546) (26.3871, -18.9698) (26.4807, -18.9844) (26.5745, -18.9985) (26.6686, -19.0119) (26.7629, -19.0248) (26.8574, -19.0371) (26.9522, -19.0489) (27.0472, -19.0601) (27.1424, -19.0707) (27.2378, -19.0808) (27.3334, -19.0903) (27.4292, -19.0993) (27.5253, -19.1078) (27.6215, -19.1157) (27.7179, -19.123) (27.8145, -19.1298) (27.9113, -19.1361) (28.0082, -19.1419) (28.1054, -19.1471) (28.2027, -19.1518) (28.3002, -19.156) (28.3979, -19.1596) (28.4957, -19.1627) (28.5937, -19.1653) (28.6918, -19.1674) (28.7901, -19.169) (28.8886, -19.1701) (28.9872, -19.1706) (29.0859, -19.1707) (29.165, -19.1703) (29.2244, -19.1698) (29.2641, -19.1693) (29.2839, -19.1691) knots 0 0 0 0 0 0 0.01428571 0.02857143 0.04285714 0.05714286 0.07142857 0.08571429 0.1 0.11428571 0.12857143 0.14285714 0.15714286 0.17142857 0.18571429 0.2 0.21428571 0.22857143 0.24285714 0.25714286 0.27142857 0.28571429 0.3 0.31428571 0.32857143 0.34285714 0.35714286 0.37142857 0.38571429 0.4 0.41428571 0.42857143 0.44285714 0.45714286 0.47142857 0.48571429 0.5 0.51428571 0.52857143 0.54285714 0.55714286 0.57142857 0.58571429 0.6 0.61428571 0.62857143 0.64285714 0.65714286 0.67142857 0.68571429 0.7 0.71428571 0.72857143 0.74285714 0.75714286 0.77142857 0.78571429 0.8 0.81428571 0.82857143 0.84285714 0.85714286 0.87142857 0.88571429 0.9 0.91428571 0.92857143 0.94285714 0.95714286 0.97142857 0.98571429 1 1 1 1 1 1
  arc A22 (29.2839, -19.1691) -> (31.2429, -15.776) centre (0, 0) ccw
  spline S11 degree 5 poles (31.2429, -15.776) (31.2332, -15.7587) (31.2137, -15.7242) (31.1845, -15.6725) (31.1452, -15.6038) (31.0958, -15.5183) (31.0461, -15.4332) (30.9959, -15.3485) (30.9454, -15.2641) (30.8945, -15.1802) (30.8433, -15.0966) (30.7916, -15.0135) (30.7397, -14.9307) (30.6873, -14.8484) (30.6346, -14.7664) (30.5815, -14.6849) (30.528, -14.6038) (30.4742, -14.5231) (30.42, -14.4429) (30.3654, -14.3631) (30.3104, -14.2837) (30.2551, -14.2048) (30.1994, -14.1263) (30.1434, -14.0482) (30.0869, -13.9706) (30.0301, -13.8935) (29.9729, -13.8168) (29.9154, -13.7406) (29.8574, -13.6649) (29.7991, -13.5897) (29.7404, -13.515) (29.6813, -13.4407) (29.6219, -13.367) (29.5621, -13.2937) (29.5019, -13.221) (29.4413, -13.1488) (29.3803, -13.0771) (29.3189, -13.0059) (29.2572, -12.9353) (29.195, -12.8653) (29.1325, -12.7958) (29.0696, -12.7268) (29.0063, -12.6585) (28.9426, -12.5907) (28.8784, -12.5236) (28.8139, -12.457) (28.749, -12.3911) (28.6837, -12.3257) (28.618, -12.261) (28.5519, -12.1969) (28.4853, -12.1335) (28.4183, -12.0708) (28.3509, -12.0089) (28.283, -11.9477) (28.2146, -11.8873) (28.1458, -11.8276) (28.0767, -11.7686) (28.0071, -11.7102) (27.9371, -11.6526) (27.8667, -11.5957) (27.7957, -11.5399) (27.7241, -11.4852) (27.6518, -11.4317) (27.5789, -11.3795) (27.5053, -11.3285) (27.4314, -11.2782) (27.3571, -11.2286) (27.2826, -11.1795) (27.2076, -11.1314) (27.1319, -11.0848) (27.055, -11.0409) (26.992, -11.0086) (26.9438, -10.9864) (26.9112, -10.9726) (26.8948, -10.9659) knots -1 -1 -1 -1 -1 -1 -0.98571429 -0.97142857 -0.95714286 -0.94285714 -0.92857143 -0.91428571 -0.9 -0.88571429 -0.87142857 -0.85714286 -0.84285714 -0.82857143 -0.81428571 -0.8 -0.78571429 -0.77142857 -0.75714286 -0.74285714 -0.72857143 -0.71428571 -0.7 -0.68571429 -0.67142857 -0.65714286 -0.64285714 -0.62857143 -0.61428571 -0.6 -0.58571429 -0.57142857 -0.55714286 -0.54285714 -0.52857143 -0.51428571 -0.5 -0.48571429 -0.47142857 -0.45714286 -0.44285714 -0.42857143 -0.41428571 -0.4 -0.38571429 -0.37142857 -0.35714286 -0.34285714 -0.32857143 -0.31428571 -0.3 -0.28571429 -0.27142857 -0.25714286 -0.24285714 -0.22857143 -0.21428571 -0.2 -0.18571429 -0.17142857 -0.15714286 -0.14285714 -0.12857143 -0.11428571 -0.1 -0.08571429 -0.07142857 -0.05714286 -0.04285714 -0.02857143 -0.01428571 0 0 0 0 0 0
  line L11 (26.8948, -10.9659) -> (23.0842, -9.411)
  arc A23 (22.5216, -8.145) -> (23.0842, -9.411) centre (23.462, -8.4851) ccw
  arc A24 (22.5216, -8.145) -> (23.5768, -4.207) centre (0, 0) ccw
  arc A25 (24.697, -3.3919) -> (23.5768, -4.207) centre (24.5612, -4.3827) ccw
  line L12 (24.697, -3.3919) -> (28.7745, -3.9507)
  spline S12 degree 5 poles (28.7745, -3.9507) (28.792, -3.9531) (28.8272, -3.9574) (28.88, -3.9623) (28.9507, -3.9658) (29.0393, -3.9662) (29.1282, -3.9638) (29.2172, -3.9595) (29.3063, -3.9544) (29.3954, -3.9485) (29.4846, -3.9419) (29.5738, -3.9345) (29.663, -3.9257) (29.7523, -3.9156) (29.8417, -3.904) (29.9311, -3.8911) (30.0205, -3.8771) (30.11, -3.8622) (30.1994, -3.8464) (30.2888, -3.8299) (30.3782, -3.8126) (30.4676, -3.7945) (30.557, -3.7754) (30.6464, -3.7555) (30.7357, -3.7347) (30.8251, -3.7131) (30.9144, -3.6907) (31.0037, -3.6675) (31.0929, -3.6435) (31.1821, -3.6189) (31.2712, -3.5935) (31.3604, -3.5674) (31.4494, -3.5406) (31.5384, -3.5131) (31.6274, -3.4848) (31.7163, -3.4559) (31.8051, -3.4263) (31.8939, -3.396) (31.9826, -3.365) (32.0713, -3.3335) (32.1598, -3.3012) (32.2484, -3.2683) (32.3368, -3.2348) (32.4251, -3.2007) (32.5134, -3.1659) (32.6016, -3.1305) (32.6897, -3.0945) (32.7778, -3.0579) (32.8657, -3.0207) (32.9536, -2.9829) (33.0413, -2.9445) (33.129, -2.9056) (33.2166, -2.866) (33.3041, -2.8259) (33.3915, -2.7852) (33.4787, -2.7439) (33.5659, -2.7021) (33.653, -2.6597) (33.7399, -2.6167) (33.8268, -2.5732) (33.9135, -2.5292) (34.0002, -2.4846) (34.0867, -2.4394) (34.1731, -2.3938) (34.2594, -2.3476) (34.3455, -2.3008) (34.4316, -2.2536) (34.5175, -2.2058) (34.6033, -2.1575) (34.6889, -2.1087) (34.7745, -2.0593) (34.8428, -2.0194) (34.894, -1.9893) (34.9281, -1.9691) (34.9451, -1.959) knots 0 0 0 0 0 0 0.01428571 0.02857143 0.04285714 0.05714286 0.07142857 0.08571429 0.1 0.11428571 0.12857143 0.14285714 0.15714286 0.17142857 0.18571429 0.2 0.21428571 0.22857143 0.24285714 0.25714286 0.27142857 0.28571429 0.3 0.31428571 0.32857143 0.34285714 0.35714286 0.37142857 0.38571429 0.4 0.41428571 0.42857143 0.44285714 0.45714286 0.47142857 0.48571429 0.5 0.51428571 0.52857143 0.54285714 0.55714286 0.57142857 0.58571429 0.6 0.61428571 0.62857143 0.64285714 0.65714286 0.67142857 0.68571429 0.7 0.71428571 0.72857143 0.74285714 0.75714286 0.77142857 0.78571429 0.8 0.81428571 0.82857143 0.84285714 0.85714286 0.87142857 0.88571429 0.9 0.91428571 0.92857143 0.94285714 0.95714286 0.97142857 0.98571429 1 1 1 1 1 1
  arc A26 (34.9451, -1.959) -> (34.9451, 1.959) centre (0, 0) ccw
  spline S13 degree 5 poles (34.9451, 1.959) (34.9281, 1.9691) (34.894, 1.9893) (34.8428, 2.0194) (34.7745, 2.0593) (34.6889, 2.1087) (34.6033, 2.1575) (34.5175, 2.2058) (34.4316, 2.2536) (34.3455, 2.3008) (34.2594, 2.3476) (34.1731, 2.3938) (34.0867, 2.4394) (34.0002, 2.4846) (33.9135, 2.5292) (33.8268, 2.5732) (33.7399, 2.6167) (33.653, 2.6597) (33.5659, 2.7021) (33.4787, 2.7439) (33.3915, 2.7852) (33.3041, 2.8259) (33.2166, 2.866) (33.129, 2.9056) (33.0413, 2.9445) (32.9536, 2.9829) (32.8657, 3.0207) (32.7778, 3.0579) (32.6897, 3.0945) (32.6016, 3.1305) (32.5134, 3.1659) (32.4251, 3.2007) (32.3368, 3.2348) (32.2484, 3.2683) (32.1598, 3.3012) (32.0713, 3.3335) (31.9826, 3.365) (31.8939, 3.396) (31.8051, 3.4263) (31.7163, 3.4559) (31.6274, 3.4848) (31.5384, 3.5131) (31.4494, 3.5406) (31.3604, 3.5674) (31.2712, 3.5935) (31.1821, 3.6189) (31.0929, 3.6435) (31.0037, 3.6675) (30.9144, 3.6907) (30.8251, 3.7131) (30.7357, 3.7347) (30.6464, 3.7555) (30.557, 3.7754) (30.4676, 3.7945) (30.3782, 3.8126) (30.2888, 3.8299) (30.1994, 3.8464) (30.11, 3.8622) (30.0205, 3.8771) (29.9311, 3.8911) (29.8417, 3.904) (29.7523, 3.9156) (29.663, 3.9257) (29.5738, 3.9345) (29.4846, 3.9419) (29.3954, 3.9485) (29.3063, 3.9544) (29.2172, 3.9595) (29.1282, 3.9638) (29.0393, 3.9662) (28.9507, 3.9658) (28.88, 3.9623) (28.8272, 3.9574) (28.792, 3.9531) (28.7745, 3.9507) knots -1 -1 -1 -1 -1 -1 -0.98571429 -0.97142857 -0.95714286 -0.94285714 -0.92857143 -0.91428571 -0.9 -0.88571429 -0.87142857 -0.85714286 -0.84285714 -0.82857143 -0.81428571 -0.8 -0.78571429 -0.77142857 -0.75714286 -0.74285714 -0.72857143 -0.71428571 -0.7 -0.68571429 -0.67142857 -0.65714286 -0.64285714 -0.62857143 -0.61428571 -0.6 -0.58571429 -0.57142857 -0.55714286 -0.54285714 -0.52857143 -0.51428571 -0.5 -0.48571429 -0.47142857 -0.45714286 -0.44285714 -0.42857143 -0.41428571 -0.4 -0.38571429 -0.37142857 -0.35714286 -0.34285714 -0.32857143 -0.31428571 -0.3 -0.28571429 -0.27142857 -0.25714286 -0.24285714 -0.22857143 -0.21428571 -0.2 -0.18571429 -0.17142857 -0.15714286 -0.14285714 -0.12857143 -0.11428571 -0.1 -0.08571429 -0.07142857 -0.05714286 -0.04285714 -0.02857143 -0.01428571 0 0 0 0 0 0
  line L13 (28.7745, 3.9507) -> (24.697, 3.3919)
  arc A27 (23.5768, 4.207) -> (24.697, 3.3919) centre (24.5612, 4.3827) ccw
  arc A28 (23.5768, 4.207) -> (22.5216, 8.145) centre (0, 0) ccw
  arc A29 (23.0842, 9.411) -> (22.5216, 8.145) centre (23.462, 8.4851) ccw
  line L14 (23.0842, 9.411) -> (26.8948, 10.9659)
  spline S14 degree 5 poles (26.8948, 10.9659) (26.9112, 10.9726) (26.9438, 10.9864) (26.992, 11.0086) (27.055, 11.0409) (27.1319, 11.0848) (27.2076, 11.1314) (27.2826, 11.1795) (27.3571, 11.2286) (27.4314, 11.2782) (27.5053, 11.3285) (27.5789, 11.3795) (27.6518, 11.4317) (27.7241, 11.4852) (27.7957, 11.5399) (27.8667, 11.5957) (27.9371, 11.6526) (28.0071, 11.7102) (28.0767, 11.7686) (28.1458, 11.8276) (28.2146, 11.8873) (28.283, 11.9477) (28.3509, 12.0089) (28.4183, 12.0708) (28.4853, 12.1335) (28.5519, 12.1969) (28.618, 12.261) (28.6837, 12.3257) (28.749, 12.3911) (28.8139, 12.457) (28.8784, 12.5236) (28.9426, 12.5907) (29.0063, 12.6585) (29.0696, 12.7268) (29.1325, 12.7958) (29.195, 12.8653) (29.2572, 12.9353) (29.3189, 13.0059) (29.3803, 13.0771) (29.4413, 13.1488) (29.5019, 13.221) (29.5621, 13.2937) (29.6219, 13.367) (29.6813, 13.4407) (29.7404, 13.515) (29.7991, 13.5897) (29.8574, 13.6649) (29.9154, 13.7406) (29.9729, 13.8168) (30.0301, 13.8935) (30.0869, 13.9706) (30.1434, 14.0482) (30.1994, 14.1263) (30.2551, 14.2048) (30.3104, 14.2837) (30.3654, 14.3631) (30.42, 14.4429) (30.4742, 14.5231) (30.528, 14.6038) (30.5815, 14.6849) (30.6346, 14.7664) (30.6873, 14.8484) (30.7397, 14.9307) (30.7916, 15.0135) (30.8433, 15.0966) (30.8945, 15.1802) (30.9454, 15.2641) (30.9959, 15.3485) (31.0461, 15.4332) (31.0958, 15.5183) (31.1452, 15.6038) (31.1845, 15.6725) (31.2137, 15.7242) (31.2332, 15.7587) (31.2429, 15.776) knots 0 0 0 0 0 0 0.01428571 0.02857143 0.04285714 0.05714286 0.07142857 0.08571429 0.1 0.11428571 0.12857143 0.14285714 0.15714286 0.17142857 0.18571429 0.2 0.21428571 0.22857143 0.24285714 0.25714286 0.27142857 0.28571429 0.3 0.31428571 0.32857143 0.34285714 0.35714286 0.37142857 0.38571429 0.4 0.41428571 0.42857143 0.44285714 0.45714286 0.47142857 0.48571429 0.5 0.51428571 0.52857143 0.54285714 0.55714286 0.57142857 0.58571429 0.6 0.61428571 0.62857143 0.64285714 0.65714286 0.67142857 0.68571429 0.7 0.71428571 0.72857143 0.74285714 0.75714286 0.77142857 0.78571429 0.8 0.81428571 0.82857143 0.84285714 0.85714286 0.87142857 0.88571429 0.9 0.91428571 0.92857143 0.94285714 0.95714286 0.97142857 0.98571429 1 1 1 1 1 1
  arc A30 (31.2429, 15.776) -> (29.2839, 19.1691) centre (0, 0) ccw
  spline S15 degree 5 poles (29.2839, 19.1691) (29.2641, 19.1693) (29.2244, 19.1698) (29.165, 19.1703) (29.0859, 19.1707) (28.9872, 19.1706) (28.8886, 19.1701) (28.7901, 19.169) (28.6918, 19.1674) (28.5937, 19.1653) (28.4957, 19.1627) (28.3979, 19.1596) (28.3002, 19.156) (28.2027, 19.1518) (28.1054, 19.1471) (28.0082, 19.1419) (27.9113, 19.1361) (27.8145, 19.1298) (27.7179, 19.123) (27.6215, 19.1157) (27.5253, 19.1078) (27.4292, 19.0993) (27.3334, 19.0903) (27.2378, 19.0808) (27.1424, 19.0707) (27.0472, 19.0601) (26.9522, 19.0489) (26.8574, 19.0371) (26.7629, 19.0248) (26.6686, 19.0119) (26.5745, 18.9985) (26.4807, 18.9844) (26.3871, 18.9698) (26.2937, 18.9546) (26.2006, 18.9389) (26.1078, 18.9225) (26.0152, 18.9055) (25.9229, 18.888) (25.8309, 18.8698) (25.7392, 18.851) (25.6477, 18.8316) (25.5565, 18.8116) (25.4657, 18.7909) (25.3752, 18.7696) (25.2849, 18.7477) (25.1951, 18.7251) (25.1055, 18.7018) (25.0162, 18.6779) (24.9273, 18.6534) (24.8388, 18.6282) (24.7506, 18.6022) (24.6628, 18.5756) (24.5754, 18.5481) (24.4885, 18.5199) (24.402, 18.4909) (24.3159, 18.4612) (24.2302, 18.4308) (24.1449, 18.3997) (24.06, 18.3679) (23.9755, 18.3354) (23.8917, 18.3018) (23.8085, 18.2672) (23.7261, 18.2313) (23.6444, 18.1942) (23.5634, 18.1561) (23.4829, 18.1172) (23.4028, 18.0777) (23.3231, 18.0377) (23.2439, 17.9968) (23.1657, 17.9545) (23.0891, 17.9099) (23.0297, 17.8714) (22.9864, 17.8408) (22.9581, 17.8195) (22.9441, 17.8086) knots -1 -1 -1 -1 -1 -1 -0.98571429 -0.97142857 -0.95714286 -0.94285714 -0.92857143 -0.91428571 -0.9 -0.88571429 -0.87142857 -0.85714286 -0.84285714 -0.82857143 -0.81428571 -0.8 -0.78571429 -0.77142857 -0.75714286 -0.74285714 -0.72857143 -0.71428571 -0.7 -0.68571429 -0.67142857 -0.65714286 -0.64285714 -0.62857143 -0.61428571 -0.6 -0.58571429 -0.57142857 -0.55714286 -0.54285714 -0.52857143 -0.51428571 -0.5 -0.48571429 -0.47142857 -0.45714286 -0.44285714 -0.42857143 -0.41428571 -0.4 -0.38571429 -0.37142857 -0.35714286 -0.34285714 -0.32857143 -0.31428571 -0.3 -0.28571429 -0.27142857 -0.25714286 -0.24285714 -0.22857143 -0.21428571 -0.2 -0.18571429 -0.17142857 -0.15714286 -0.14285714 -0.12857143 -0.11428571 -0.1 -0.08571429 -0.07142857 -0.05714286 -0.04285714 -0.02857143 -0.01428571 0 0 0 0 0 0
  line L15 (22.9441, 17.8086) -> (19.6923, 15.286)
  arc A31 (18.3146, 15.4318) -> (19.6923, 15.286) centre (19.0793, 16.0761) ccw
  arc A32 (18.3146, 15.4318) -> (15.4318, 18.3146) centre (0, 0) ccw
  arc A33 (15.286, 19.6923) -> (15.4318, 18.3146) centre (16.0761, 19.0793) ccw
  line L16 (15.286, 19.6923) -> (17.8086, 22.9441)
  spline S16 degree 5 poles (17.8086, 22.9441) (17.8195, 22.9581) (17.8408, 22.9864) (17.8714, 23.0297) (17.9099, 23.0891) (17.9545, 23.1657) (17.9968, 23.2439) (18.0377, 23.3231) (18.0777, 23.4028) (18.1172, 23.4829) (18.1561, 23.5634) (18.1942, 23.6444) (18.2313, 23.7261) (18.2672, 23.8085) (18.3018, 23.8917) (18.3354, 23.9755) (18.3679, 24.06) (18.3997, 24.1449) (18.4308, 24.2302) (18.4612, 24.3159) (18.4909, 24.402) (18.5199, 24.4885) (18.5481, 24.5754) (18.5756, 24.6628) (18.6022, 24.7506) (18.6282, 24.8388) (18.6534, 24.9273) (18.6779, 25.0162) (18.7018, 25.1055) (18.7251, 25.1951) (18.7477, 25.2849) (18.7696, 25.3752) (18.7909, 25.4657) (18.8116, 25.5565) (18.8316, 25.6477) (18.851, 25.7392) (18.8698, 25.8309) (18.888, 25.9229) (18.9055, 26.0152) (18.9225, 26.1078) (18.9389, 26.2006) (18.9546, 26.2937) (18.9698, 26.3871) (18.9844, 26.4807) (18.9985, 26.5745) (19.0119, 26.6686) (19.0248, 26.7629) (19.0371, 26.8574) (19.0489, 26.9522) (19.0601, 27.0472) (19.0707, 27.1424) (19.0808, 27.2378) (19.0903, 27.3334) (19.0993, 27.4292) (19.1078, 27.5253) (19.1157, 27.6215) (19.123, 27.7179) (19.1298, 27.8145) (19.1361, 27.9113) (19.1419, 28.0082) (19.1471, 28.1054) (19.1518, 28.2027) (19.156, 28.3002) (19.1596, 28.3979) (19.1627, 28.4957) (19.1653, 28.5937) (19.1674, 28.6918) (19.169, 28.7901) (19.1701, 28.8886) (19.1706, 28.9872) (19.1707, 29.0859) (19.1703, 29.165) (19.1698, 29.2244) (19.1693, 29.2641) (19.1691, 29.2839) knots 0 0 0 0 0 0 0.01428571 0.02857143 0.04285714 0.05714286 0.07142857 0.08571429 0.1 0.11428571 0.12857143 0.14285714 0.15714286 0.17142857 0.18571429 0.2 0.21428571 0.22857143 0.24285714 0.25714286 0.27142857 0.28571429 0.3 0.31428571 0.32857143 0.34285714 0.35714286 0.37142857 0.38571429 0.4 0.41428571 0.42857143 0.44285714 0.45714286 0.47142857 0.48571429 0.5 0.51428571 0.52857143 0.54285714 0.55714286 0.57142857 0.58571429 0.6 0.61428571 0.62857143 0.64285714 0.65714286 0.67142857 0.68571429 0.7 0.71428571 0.72857143 0.74285714 0.75714286 0.77142857 0.78571429 0.8 0.81428571 0.82857143 0.84285714 0.85714286 0.87142857 0.88571429 0.9 0.91428571 0.92857143 0.94285714 0.95714286 0.97142857 0.98571429 1 1 1 1 1 1
  arc A34 (19.1691, 29.2839) -> (15.776, 31.2429) centre (0, 0) ccw